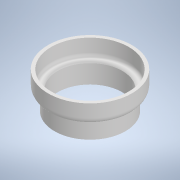
# Autodesk Inventor part: headset bearing
Saved by Autodesk Inventor 2022.2 (Build 262287000, 287)
## iProperties
Created: 2022-04-06
Part Number: headset bearing
Material: Generic
Document SubType Name: Modeling
Designer: Finn Oriwohl
Density: 1 g/cm^3
Appearance: Default
Author: Finn Oriwohl
Autodesk Inventor part; units mm, degrees
ref_plane "YZ Plane" through (0, 0, 0) normal (1, 0, 0) x (0, 1, 0)
ref_plane "XZ Plane" through (0, 0, 0) normal (0, 1, 0) x (-1, 0, 0)
ref_plane "XY Plane" through (0, 0, 0) normal (0, 0, 1) x (1, 0, 0)
sketch "Sketch1" plane through (0, 0, 0) normal (0, 0, 1) x (1, 0, 0)
  line L0 (0, 0) -> (17, 0) construction
  line L1 (20, 3) -> (20, 9)
  line L2 (17, 0) -> (17, -7.7504)
  arc A0 (17, 0) -> (20, 3) centre (17, 3) ccw
  line L3 (17, 0) -> (17, 0)
  line L4 (18, 9) -> (18, 3)
  arc A1 (17, 2) -> (18, 3) centre (17, 3) ccw
  line L5 (17, 2) -> (0, 2)
  line L6 (15, -7.7504) -> (15, 0.8352)
  line L7 (15, 0.8352) -> (15, 0.1716)
  arc A2 (17, 2) -> (15, 0.8352) centre (17.1663, -0.5851) ccw
  line L8 (18, 9) -> (20, 9)
  line L9 (17, -7.7504) -> (15, -7.7504)
  line L10 (0, 0) -> (0, 2.7427)
  point P0 (20, 0)
  point P1 (15, 0.1716)
  point P2 (17, 0)
  dimension "d0" = 9
  dimension "d1" = 3
  dimension "d3" = 17
  dimension "d4" = 3
  dimension "d5" = 2
  dimension "d9" = 2
  constraints: 22 end point, 7 point on circle, 4 vertical, 3 centre point, 3 point on line, 2 horizontal, 2 tangent, 1 parallel, 3 other
  measures "d0" distance of point (20, 0) L1.end
  measures "d1" distance of L2.start point (20, 0)
  measures "d3" distance of L0.start L2.start
  measures "d4" radius of A0
  measures "d5" radial gap between concentric circles of A0 A1
  measures "d9" distance between parallel lines of L2 L6
revolve "Revolution1" add sketch "Sketch1" angle 360 about axis through (0, 0, 0) along (0, 1, 0)
equation "\"d9\" = d5"
body "Solid1"
